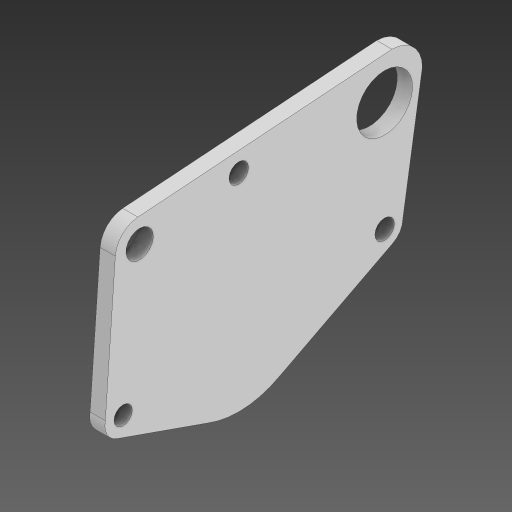
# Autodesk Inventor part: drib_lef
Saved by Autodesk Inventor 2023 (Build 270158000, 158)
## iProperties
Created: 2025-05-23
Part Number: drib_lef
Material: Типовые
Document SubType Name: Sheet Metal
Designer: daa
Density: 1 g/cm^3
Appearance: По умолчанию
Sheet Metal Rule: По умолчанию
Author: daa
Autodesk Inventor part; units mm, degrees
ref_plane "YZ Plane" through (0, 0, 0) normal (1, 0, 0) x (0, 1, 0)
ref_plane "XZ Plane" through (0, 0, 0) normal (0, 1, 0) x (-1, 0, 0)
ref_plane "XY Plane" through (0, 0, 0) normal (0, 0, 1) x (1, 0, 0)
sketch "Эскиз1" plane through (0, 0, 0) normal (1, 0, 0) x (0, 1, 0)
  circle A0 centre (25.7199, 46.7921) radius 2.25
  circle A1 centre (25.6987, 6.5017) radius 4.6
  circle A2 centre (7.6987, 6.5017) radius 1.6
  arc A3 (27.6873, 0.2956) -> (32.7199, 5.2955) centre (27.7199, 5.2955) ccw
  circle A4 centre (7.6843, 30.491) radius 14
  arc A5 (14.2267, 42.8683) -> (-1.4853, 19.9118) centre (7.6843, 30.491) ccw
  circle A6 centre (27.6987, 30.491) radius 1.6
  line L0 (7.6843, 30.491) -> (25.6987, 6.5017)
  circle A7 centre (2.6987, 49.5017) radius 1.5
  circle A8 centre (7.6987, 6.5017) radius 3
  line L1 (7.6987, 3.5017) -> (27.6873, 0.2956)
  circle A9 centre (2.6987, 49.5017) radius 3
  line L2 (-3.2958, 40.9198) -> (-5.3755, 35.5348)
  line L3 (-0.0999, 50.5825) -> (-5.3755, 35.5348)
  line L4 (-1.3769, 17.8835) -> (-4.5981, 23.7723)
  line L5 (-4.5981, 23.7723) -> (5.0667, 5.062)
  circle A10 centre (25.7199, 46.7921) radius 4
  line L6 (2.4504, 52.4914) -> (23, 51)
  line L7 (2.4504, 52.4914) -> (26.0094, 50.7816)
  line L8 (32.7199, 5.2955) -> (29.7095, 47.0795)
  point P0 (0, 0)
  point P1 (-2.3427, 0)
  point P2 (7.6843, 30.491)
  point P3 (7.6843, 30.491)
  point P4 (-4.5981, 23.7723)
  point P5 (-3.3371, 41.4181)
  point P6 (-5.3755, 35.5348)
  point P7 (5.0013, 5.1886)
  point P8 (-0.1621, 50.405)
  point P9 (3.376, 52.4242)
  dimension "d132" = 28
  dimension "d9" = 4.5
  dimension "d86" = 9.2
  dimension "d87" = 3.2
  dimension "d92" = 5
  dimension "d145" = 3.2
  dimension "d191" = 30
  dimension "d227" = 3
  dimension "d234" = 6
  dimension "d235" = 6
  dimension "d242" = 8
  constraints: 18 end point, 13 point on circle, 10 centre point, 6 coincident, 3 tangent, 5 other
  measures "d9" diameter of A0
  measures "d86" diameter of A1
  measures "d87" diameter of A2
  measures "d92" radius of A3
  measures "d145" diameter of A6
  measures "d191" distance of L0.start L0.end
  measures "d227" diameter of A7
  measures "d234" diameter of A8
  measures "d235" diameter of A9
  measures "d242" diameter of A10
extrude "Выдавливание1" add sketch "Эскиз1" along normal blind 2.5 contours A8 | A4 L3 A9 L6 L7 A10 L8 A3 L1 A8 L5 | A4 | L6 A9 | A10
equation "\"Радиус_гибки\" = Толщина"
equation "\"Ширина_просечки\" = Толщина"
equation "\"Глубина_просечки\" = 0.5 * Толщина"
equation "\"Размер_просечки\" = 4 * Толщина"
equation "\"Мин_остаток\" = 2 * Толщина"
equation "\"Радиус_перехода\" = Радиус_гибки"
equation "\"Радиус_Якоби\" = Радиус_гибки"
equation "\"Размер_зазора\" = Толщина"
equation "\"Толщина\" = 3.048"
